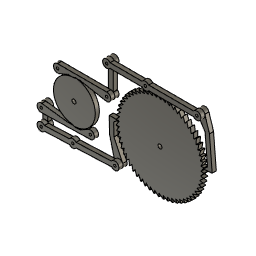
cam_driven_ratchet (Autodesk Fusion 360 design; units mm, degrees)
Autodesk Fusion 360 part; units mm, degrees
note: some values were not read from the file. Set by a fixed rule: which sketch regions a step uses.
sketch "dimensions" plane through (0, 0, 0) normal (0, 1, 0) x (1, 0, 0)
  circle A0 centre (0, 0) radius 25 construction
  line L0 (0, -25) -> (-20, -25) construction
  line L1 (0, -25) -> (40, -25) construction
  line L2 (40, -25) -> (40, -60) construction
  line L3 (40, -60) -> (87.1429, -60) construction
  line L4 (0, 25) -> (20, 25) construction
  line L5 (0, 25) -> (-40, 25) construction
  line L6 (-40, 25) -> (-40, 45) construction
  line L7 (-40, 45) -> (-1.4286, 45) construction
  line L8 (-1.4286, 45) -> (50, 45) construction
  line L9 (87.1429, -60) -> (150, -60) construction
  line L10 (50, 45) -> (50, 0) construction
  line L11 (150, -60) -> (150, 0) construction
  line L12 (150, 0) -> (50, 0) construction
  circle A1 centre (100, 0) radius 50 construction
  arc A2 (150, 0) -> (149.7261, 5.2264) centre (100, 0) ccw construction
  line L13 (100, 0) -> (150, 0) construction
  line L14 (100, 0) -> (149.7261, 5.2264) construction
  line L15 (0, 0) -> (300, 0) construction
  line L16 (0, -25) -> (0, -26) construction
  line L17 (-20, -25) -> (0, -26) construction
  line L18 (0, -26) -> (44.9579, -28.2479) construction
  line L19 (40, -25) -> (40, -28) construction
  arc A3 (39.9251, -27.9963) -> (40, -25) centre (-20, -25) ccw construction
  line L20 (-20, -25) -> (39.9251, -27.9963) construction
  line L21 (-20, -25) -> (40, -25) construction
  line L22 (40, -60) -> (40, -63) construction
  line L23 (150, -60) -> (150, -56) construction
  line L24 (40, -63) -> (150, -56) construction
  line L25 (0, 25) -> (0, 26) construction
  dimension "d4" = 20
  dimension "d5" = 40
  dimension "d6" = 35
  dimension "d7" = 47.1429
  dimension "d8" = 62.8571
  dimension "d9" = 20
  dimension "d10" = 40
  dimension "d11" = 20
  dimension "d12" = 38.5714
  dimension "d13" = 51.4286
  dimension "d14" = 50
  dimension "d25" = 100
  dimension "d173" = 6
  dimension "d185" = 1
  dimension "d190" = 3
  dimension "d191" = 2.862
  dimension "d192" = 3
  dimension "d193" = 4
  dimension "d195" = 1
  constraint coincident A0.centre L15.start
  constraint coincident A0 L0.start
  constraint horizontal L0
  constraint perpendicular L2 L3
  constraint coincident A0 L4.start
  constraint horizontal L4
  constraint perpendicular L5 L6
  constraint perpendicular L6 L7
  constraint parallel L7 L8
  constraint coincident L3.end L9.start
  constraint horizontal L3
  constraint horizontal L1
  constraint horizontal L5
  constraint tangent A0 L5
  constraint tangent A0 L1
  constraint perpendicular L9 L11
  constraint perpendicular L10 L12
  constraint midpoint L12 A1.centre
  constraint coincident L10.end A1
  constraint coincident A1.centre A2.centre
  constraint parallel L4 L15
  constraint collinear L12 L15
  constraint horizontal L9
  constraint parallel L17 L18
  constraint coincident L2 L19.end
  constraint coincident L18 L19.end
  constraint vertical L16
  constraint coincident L0.end L17.start
  constraint collinear L18 L20
  constraint perpendicular L3 L22
  constraint perpendicular L9 L23
  constraint perpendicular L4 L25
  measures "d4" distance of L0.start L0.end
  measures "d5" distance of L0.start L1.end
  measures "d6" distance of L1.end L2.end
  measures "d7" distance of L2.end L3.end
  measures "d8" distance of L3.end L9.end
  measures "d9" distance of L4.start L4.end
  measures "d10" distance of L4.start L5.end
  measures "d11" distance of L5.end L6.end
  measures "d12" distance of L6.end L7.end
  measures "d13" distance of L7.end L8.end
  measures "d14" diameter of A0
  measures "d25" diameter of A1
  measures "d173" angle of L13 L14
  measures "d185" distance of L0.start L16.end
  measures "d190" distance of L1.end L19.end
  measures "d191" angle of L20 L21
  measures "d192" distance of L2.end L22.end
  measures "d193" distance of L9.end L23.end
  measures "d195" distance of L4.start L25.end
sketch "cam" plane through (0, 0, 0) normal (0, 1, 0) x (1, 0, 0)
  circle A0 centre (0, 0) radius 2.5
  circle A1 centre (0, 0) radius 25 construction
  arc A2 (-1.3084, -24.9657) -> (0, -25) centre (0, 0) ccw construction
  line L0 (0, 0) -> (-1.3084, -24.9657) construction
  line L1 (0, 0) -> (0, -25) construction
  arc A3 (0, -26) -> (1.3607, -25.9644) centre (0, 0) ccw construction
  line L2 (0, 0) -> (0, -26) construction
  line L3 (0, 0) -> (1.3607, -25.9644) construction
  arc A4 (0, 25) -> (-1.3084, 24.9657) centre (0, 0) ccw construction
  line L4 (0, 0) -> (0, 25) construction
  line L5 (0, 0) -> (-1.3084, 24.9657) construction
  arc A5 (1.3607, 25.9644) -> (0, 26) centre (0, 0) ccw construction
  line L6 (0, 0) -> (1.3607, 25.9644) construction
  line L7 (0, 0) -> (0, 26) construction
  line L8 (-1.3084, 24.9657) -> (1.3607, 25.9644)
  line L9 (-1.3084, -24.9657) -> (1.3607, -25.9644)
  arc A6 (1.3607, -25.9644) -> (1.3607, 25.9644) centre (0, 0) ccw
  arc A7 (-1.3084, 24.9657) -> (-1.3084, -24.9657) centre (0, 0) ccw
  point P0 (0, -26)
  point P1 (0, -25)
  point P2 (0, 25)
  point P3 (0, 26)
  dimension "d194" = 5
  dimension "d196" = 3
  dimension "d197" = 3
  dimension "d198" = 3
  dimension "d199" = 3
  constraint coincident A0.centre A1.centre
  constraint coincident P1 A2.end
  constraint coincident P0 A3.start
  constraint coincident P2 A4.start
  constraint coincident P3 A5.end
  measures "d194" diameter of A0
  measures "d196" angle of L0 L1
  measures "d197" angle of L2 L3
  measures "d198" angle of L4 L5
  measures "d199" angle of L6 L7
sketch "arms" plane through (0, 0, 0) normal (0, 1, 0) x (1, 0, 0)
  circle A0 centre (20, 25) radius 1.5
  circle A1 centre (20, 25) radius 5
  circle A2 centre (-20, -25) radius 1.5
  circle A3 centre (-20, -25) radius 5
  circle A4 centre (-40, 25) radius 1.5
  circle A5 centre (-40, 45) radius 1.5
  circle A6 centre (-1.4286, 45) radius 1.5
  circle A7 centre (50, 45) radius 1.5
  circle A8 centre (40, -25) radius 1.5
  circle A9 centre (40, -60) radius 1.5
  circle A10 centre (87.1429, -60) radius 1.5
  circle A11 centre (150, -60) radius 1.5
  circle A12 centre (-40, 25) radius 5
  circle A13 centre (-40, 45) radius 5
  circle A14 centre (-1.4286, 45) radius 5
  circle A15 centre (50, 45) radius 5
  circle A16 centre (40, -25) radius 5
  circle A17 centre (40, -60) radius 5
  circle A18 centre (87.1429, -60) radius 5
  circle A19 centre (150, -60) radius 5
  line L0 (-1.3084, -24.9657) -> (-7.3084, -24.9657)
  line L1 (-7.3084, -24.9657) -> (-18.0426, -20.3991)
  line L2 (-20, -30) -> (40, -30)
  line L3 (20, 30) -> (-40, 30)
  line L4 (7.3607, -25.9644) -> (39.0888, -20.0837)
  line L5 (37, -60) -> (37, -25)
  line L6 (43, -60) -> (43, -25)
  line L7 (40, -63) -> (150, -63)
  line L8 (-1.3084, 24.9657) -> (-7.3084, 24.9657)
  line L9 (7.3607, 25.9644) -> (17.6839, 20.5688)
  line L10 (-7.3084, 24.9657) -> (-39.2405, 20.058)
  line L11 (1.3607, -25.9644) -> (7.3607, -25.9644)
  line L12 (1.3607, 25.9644) -> (7.3607, 25.9644)
  line L13 (-1.3084, -24.9657) -> (1.3607, -25.9644)
  line L14 (-1.3084, 24.9657) -> (1.3607, 25.9644)
  line L15 (-40, 25) -> (-43, 25) construction
  line L16 (-40, 25) -> (-37, 25) construction
  line L17 (-40, 45) -> (-43, 45) construction
  line L18 (-40, 45) -> (-37, 45) construction
  line L19 (-40, 45) -> (-40, 42) construction
  line L20 (-40, 45) -> (-40, 48) construction
  line L21 (50, 45) -> (50, 42) construction
  line L22 (50, 45) -> (50, 48) construction
  line L23 (40, -25) -> (43, -25) construction
  line L24 (40, -25) -> (37, -25) construction
  line L25 (40, -60) -> (37, -60) construction
  line L26 (40, -60) -> (43, -60) construction
  line L27 (40, -60) -> (40, -57) construction
  line L28 (40, -60) -> (40, -63) construction
  line L29 (150, -60) -> (150, -63) construction
  line L30 (150, -60) -> (150, -57) construction
  line L31 (150, -57) -> (40, -57)
  line L32 (-37, 25) -> (-37, 45)
  line L33 (-43, 25) -> (-43, 45)
  line L34 (-40, 42) -> (50, 42)
  line L35 (-40, 48) -> (50, 48)
  point P0 (40, -25)
  point P1 (-40, 25)
  point P2 (-40, 45)
  point P3 (40, -60)
  point P4 (150, -60)
  point P5 (50, 45)
  point P6 (-20, -25)
  point P7 (20, 25)
  point P8 (87.1429, -60)
  point P9 (-1.4286, 45)
  point P10 (-1.3084, 24.9657)
  point P11 (-1.3084, -24.9657)
  dimension "d37" = 3
  dimension "d38" = 10
  dimension "d39" = 3
  dimension "d40" = 10
  dimension "d41" = 3
  dimension "d42" = 3
  dimension "d43" = 3
  dimension "d44" = 3
  dimension "d45" = 3
  dimension "d46" = 3
  dimension "d47" = 3
  dimension "d48" = 3
  dimension "d49" = 10
  dimension "d50" = 10
  dimension "d51" = 10
  dimension "d52" = 10
  dimension "d53" = 10
  dimension "d54" = 10
  dimension "d55" = 10
  dimension "d56" = 10
  dimension "d57" = 6
  dimension "d149" = 6
  dimension "d170" = 6
  dimension "d171" = 6
  dimension "d200" = 3
  dimension "d201" = 3
  dimension "d203" = 3
  dimension "d204" = 3
  dimension "d205" = 3
  dimension "d206" = 3
  dimension "d207" = 3
  dimension "d208" = 3
  dimension "d209" = 3
  dimension "d210" = 3
  dimension "d211" = 3
  dimension "d212" = 3
  dimension "d213" = 3
  dimension "d214" = 3
  dimension "d215" = 3
  dimension "d216" = 3
  constraint coincident P7 A0.centre
  constraint concentric A0 A1
  constraint coincident P6 A2.centre
  constraint concentric A2 A3
  constraint coincident P1 A4.centre
  constraint coincident P2 A5.centre
  constraint coincident P9 A6.centre
  constraint coincident P5 A7.centre
  constraint coincident P0 A8.centre
  constraint coincident P3 A9.centre
  constraint coincident P8 A10.centre
  constraint coincident P4 A11.centre
  constraint concentric A4 A12
  constraint concentric A5 A13
  constraint concentric A8 A16
  constraint concentric A9 A17
  constraint concentric A11 A19
  constraint coincident A3 L1.end
  constraint tangent A3 L1
  constraint coincident A3 L2.start
  constraint coincident A16 L2.end
  constraint tangent A16 L2
  constraint horizontal L2
  constraint coincident A1 L3.start
  constraint coincident A12 L3.end
  constraint tangent A12 L3
  constraint parallel L2 L3
  constraint coincident A16 L4.end
  constraint tangent A16 L4
  constraint perpendicular L2 L5
  constraint perpendicular L2 L6
  constraint horizontal L7
  constraint horizontal L8
  constraint coincident A1 L9.end
  constraint tangent A1 L9
  constraint coincident A12 L10.end
  constraint tangent A12 L10
  constraint coincident L11.start L13.end
  constraint horizontal L11
  constraint coincident L4.start L11.end
  constraint coincident L12.start L14.end
  constraint horizontal L12
  constraint coincident L9.start L12.end
  constraint coincident P10 L8.start
  constraint coincident P11 L0.start
  constraint horizontal L0
  constraint parallel L3 L15
  constraint parallel L15 L16
  constraint horizontal L18
  constraint perpendicular L18 L19
  constraint perpendicular L18 L20
  constraint vertical L21
  constraint parallel L21 L22
  constraint perpendicular L6 L23
  constraint parallel L23 L24
  constraint perpendicular L5 L25
  constraint parallel L25 L26
  constraint perpendicular L26 L27
  constraint perpendicular L26 L28
  constraint coincident L5.start L25.end
  constraint coincident L5.end L24.end
  constraint coincident L6.end L23.end
  constraint coincident L6.start L26.end
  constraint coincident L7.start L28.end
  constraint vertical L29
  constraint parallel L29 L30
  constraint coincident L7.end L29.end
  constraint perpendicular L17 L33
  measures "d37" diameter of A0
  measures "d38" diameter of A1
  measures "d39" diameter of A2
  measures "d40" diameter of A3
  measures "d41" diameter of A4
  measures "d42" diameter of A5
  measures "d43" diameter of A6
  measures "d44" diameter of A7
  measures "d45" diameter of A8
  measures "d46" diameter of A9
  measures "d47" diameter of A10
  measures "d48" diameter of A11
  measures "d49" diameter of A12
  measures "d50" diameter of A13
  measures "d51" diameter of A14
  measures "d52" diameter of A15
  measures "d53" diameter of A16
  measures "d54" diameter of A17
  measures "d55" diameter of A18
  measures "d56" diameter of A19
  measures "d57" distance of P11 L0.end
  measures "d149" distance of P10 L8.end
  measures "d170" distance of L11.start L4.start
  measures "d171" distance of L12.start L9.start
  measures "d200" distance of P1 L15.end
  measures "d201" distance of P1 L16.end
  measures "d203" distance of P2 L17.end
  measures "d204" distance of P2 L18.end
  measures "d205" distance of P2 L19.end
  measures "d206" distance of P2 L20.end
  measures "d207" distance of P5 L21.end
  measures "d208" distance of P5 L22.end
  measures "d209" distance of P0 L6.end
  measures "d210" distance of P0 L5.end
  measures "d211" distance of P3 L5.start
  measures "d212" distance of P3 L6.start
  measures "d213" distance of P3 L27.end
  measures "d214" distance of P3 L7.start
  measures "d215" distance of P4 L7.end
  measures "d216" distance of P4 L30.end
sketch "pawls" plane through (0, 0, 0) normal (0, 1, 0) x (1, 0, 0)
  circle A0 centre (150, -60) radius 5
  circle A1 centre (150, -60) radius 1.5
  circle A2 centre (50, 45) radius 5
  circle A3 centre (50, 45) radius 1.5
  circle A4 centre (100, 0) radius 50 construction
  arc A5 (149.9315, -2.6168) -> (150, 0) centre (100, 0) ccw construction
  line L0 (100, 0) -> (149.9315, -2.6168) construction
  line L1 (100, 0) -> (150, 0) construction
  line L2 (149.9315, -2.6168) -> (153.9292, -2.7526)
  line L3 (153.9292, -2.7526) -> (160.9251, -2.9902)
  line L4 (153.9292, -2.7526) -> (153.8273, -5.7508) construction
  line L5 (149.9315, -2.6168) -> (153.8273, -5.7508)
  line L6 (153.8273, -5.7508) -> (155.3857, -7.0045)
  line L7 (160.9251, -2.9902) -> (159.5675, -42.9671)
  line L8 (159.5675, -42.9671) -> (154.8409, -61.2514)
  line L9 (159.5675, -42.9671) -> (148.1015, -42.5777) construction
  line L10 (155.3857, -7.0045) -> (154.1706, -42.7838)
  line L11 (154.1706, -42.7838) -> (145.6704, -57.499)
  line L12 (100, 0) -> (50, 0) construction
  line L13 (50, 0) -> (46, 0)
  line L14 (46, 0) -> (39, 0)
  line L15 (39, 0) -> (39, 20)
  line L16 (46, 0) -> (46, 3) construction
  line L17 (39, 20) -> (66.1936, 20) construction
  line L18 (50, 0) -> (46, 3)
  line L19 (44.4, 20) -> (54.572, 42.9759)
  line L20 (39, 20) -> (45.1321, 46.1419)
  line L21 (46, 3) -> (44.4, 4.2)
  line L22 (44.4, 4.2) -> (44.4, 20)
  dimension "d156" = 3
  dimension "d157" = 4
  dimension "d158" = 7
  dimension "d159" = 3
  dimension "d160" = 2
  dimension "d161" = 40
  dimension "d164" = 7
  dimension "d165" = 20
  dimension "d166" = 3
  dimension "d172" = 2
  dimension "d217" = 4
  constraint coincident A4 A5.end
  constraint coincident A4.centre A5.centre
  constraint parallel L2 L3
  constraint perpendicular L3 L4
  constraint parallel L5 L6
  constraint perpendicular L3 L7
  constraint coincident A0 L8.end
  constraint tangent A0 L8
  constraint perpendicular L7 L9
  constraint coincident L9 L10.end
  constraint perpendicular L9 L10
  constraint coincident A0 L11.end
  constraint tangent A0 L11
  constraint perpendicular L14 L15
  constraint perpendicular L14 L16
  constraint perpendicular L15 L17
  constraint coincident L17 L19.start
  constraint coincident A2 L19.end
  constraint tangent A2 L19
  constraint coincident A2 L20.end
  constraint tangent A2 L20
  constraint perpendicular L17 L22
  constraint coincident L19.start L22.end
  constraint horizontal L12
  constraint collinear L12 L13
  constraint coincident A4 L12.end
  constraint collinear L18 L21
  constraint horizontal L14
  constraint horizontal L1
  measures "d156" angle of L0 L1
  measures "d157" distance of A5.start L2.end
  measures "d158" distance of L2.end L3.end
  measures "d159" distance of L2.end L4.end
  measures "d160" distance of L4.end L6.end
  measures "d161" distance of L3.end L7.end
  measures "d164" distance of L13.end L14.end
  measures "d165" distance of L14.end L15.end
  measures "d166" distance of L13.end L16.end
  measures "d172" distance of L16.end L21.end
  measures "d217" distance of L12.end L13.end
sketch "wheel" plane through (0, 0, 0) normal (0, 1, 0) x (1, 0, 0)
  circle A0 centre (100, 0) radius 50 construction
  arc A1 (100, -50) -> (105.2264, -49.7261) centre (100, 0) ccw construction
  line L0 (100, 0) -> (100, -50) construction
  line L1 (100, 0) -> (105.2264, -49.7261) construction
  line L2 (100, -50) -> (100, -54)
  line L3 (100, -54) -> (105.2264, -49.7261)
  line L4 (105.6445, -53.7042) -> (110.3956, -48.9074)
  line L5 (105.2264, -49.7261) -> (105.6445, -53.7042)
  line L6 (111.2272, -52.82) -> (115.4508, -47.5528)
  line L7 (110.3956, -48.9074) -> (111.2272, -52.82)
  line L8 (116.6869, -51.3571) -> (120.3368, -45.6773)
  line L9 (115.4508, -47.5528) -> (116.6869, -51.3571)
  line L10 (121.9638, -49.3315) -> (125, -43.3013)
  line L11 (120.3368, -45.6773) -> (121.9638, -49.3315)
  line L12 (127, -46.7654) -> (129.3893, -40.4508)
  line L13 (125, -43.3013) -> (127, -46.7654)
  line L14 (131.7404, -43.6869) -> (133.4565, -37.1572)
  line L15 (129.3893, -40.4508) -> (131.7404, -43.6869)
  line L16 (136.1331, -40.1298) -> (137.1572, -33.4565)
  line L17 (133.4565, -37.1572) -> (136.1331, -40.1298)
  line L18 (140.1298, -36.1331) -> (140.4508, -29.3893)
  line L19 (137.1572, -33.4565) -> (140.1298, -36.1331)
  line L20 (143.6869, -31.7404) -> (143.3013, -25)
  line L21 (140.4508, -29.3893) -> (143.6869, -31.7404)
  line L22 (146.7654, -27) -> (145.6773, -20.3368)
  line L23 (143.3013, -25) -> (146.7654, -27)
  line L24 (149.3315, -21.9638) -> (147.5528, -15.4508)
  line L25 (145.6773, -20.3368) -> (149.3315, -21.9638)
  line L26 (151.3571, -16.6869) -> (148.9074, -10.3956)
  line L27 (147.5528, -15.4508) -> (151.3571, -16.6869)
  line L28 (152.82, -11.2272) -> (149.7261, -5.2264)
  line L29 (148.9074, -10.3956) -> (152.82, -11.2272)
  line L30 (153.7042, -5.6445) -> (150, 0)
  line L31 (149.7261, -5.2264) -> (153.7042, -5.6445)
  line L32 (154, 0) -> (149.7261, 5.2264)
  line L33 (150, 0) -> (154, 0)
  line L34 (153.7042, 5.6445) -> (148.9074, 10.3956)
  line L35 (149.7261, 5.2264) -> (153.7042, 5.6445)
  line L36 (152.82, 11.2272) -> (147.5528, 15.4508)
  line L37 (148.9074, 10.3956) -> (152.82, 11.2272)
  line L38 (151.3571, 16.6869) -> (145.6773, 20.3368)
  line L39 (147.5528, 15.4508) -> (151.3571, 16.6869)
  line L40 (149.3315, 21.9638) -> (143.3013, 25)
  line L41 (145.6773, 20.3368) -> (149.3315, 21.9638)
  line L42 (146.7654, 27) -> (140.4508, 29.3893)
  line L43 (143.3013, 25) -> (146.7654, 27)
  line L44 (143.6869, 31.7404) -> (137.1572, 33.4565)
  line L45 (140.4508, 29.3893) -> (143.6869, 31.7404)
  line L46 (140.1298, 36.1331) -> (133.4565, 37.1572)
  line L47 (137.1572, 33.4565) -> (140.1298, 36.1331)
  line L48 (136.1331, 40.1298) -> (129.3893, 40.4508)
  line L49 (133.4565, 37.1572) -> (136.1331, 40.1298)
  line L50 (131.7404, 43.6869) -> (125, 43.3013)
  line L51 (129.3893, 40.4508) -> (131.7404, 43.6869)
  line L52 (127, 46.7654) -> (120.3368, 45.6773)
  line L53 (125, 43.3013) -> (127, 46.7654)
  line L54 (121.9638, 49.3315) -> (115.4508, 47.5528)
  line L55 (120.3368, 45.6773) -> (121.9638, 49.3315)
  line L56 (116.6869, 51.3571) -> (110.3956, 48.9074)
  line L57 (115.4508, 47.5528) -> (116.6869, 51.3571)
  line L58 (111.2272, 52.82) -> (105.2264, 49.7261)
  line L59 (110.3956, 48.9074) -> (111.2272, 52.82)
  line L60 (105.6445, 53.7042) -> (100, 50)
  line L61 (105.2264, 49.7261) -> (105.6445, 53.7042)
  line L62 (100, 54) -> (94.7736, 49.7261)
  line L63 (100, 50) -> (100, 54)
  line L64 (94.3555, 53.7042) -> (89.6044, 48.9074)
  line L65 (94.7736, 49.7261) -> (94.3555, 53.7042)
  line L66 (88.7728, 52.82) -> (84.5492, 47.5528)
  line L67 (89.6044, 48.9074) -> (88.7728, 52.82)
  line L68 (83.3131, 51.3571) -> (79.6632, 45.6773)
  line L69 (84.5492, 47.5528) -> (83.3131, 51.3571)
  line L70 (78.0362, 49.3315) -> (75, 43.3013)
  line L71 (79.6632, 45.6773) -> (78.0362, 49.3315)
  line L72 (73, 46.7654) -> (70.6107, 40.4508)
  line L73 (75, 43.3013) -> (73, 46.7654)
  line L74 (68.2596, 43.6869) -> (66.5435, 37.1572)
  line L75 (70.6107, 40.4508) -> (68.2596, 43.6869)
  line L76 (63.8669, 40.1298) -> (62.8428, 33.4565)
  line L77 (66.5435, 37.1572) -> (63.8669, 40.1298)
  line L78 (59.8702, 36.1331) -> (59.5492, 29.3893)
  line L79 (62.8428, 33.4565) -> (59.8702, 36.1331)
  line L80 (56.3131, 31.7404) -> (56.6987, 25)
  line L81 (59.5492, 29.3893) -> (56.3131, 31.7404)
  line L82 (53.2346, 27) -> (54.3227, 20.3368)
  line L83 (56.6987, 25) -> (53.2346, 27)
  line L84 (50.6685, 21.9638) -> (52.4472, 15.4508)
  line L85 (54.3227, 20.3368) -> (50.6685, 21.9638)
  line L86 (48.6429, 16.6869) -> (51.0926, 10.3956)
  line L87 (52.4472, 15.4508) -> (48.6429, 16.6869)
  line L88 (47.18, 11.2272) -> (50.2739, 5.2264)
  line L89 (51.0926, 10.3956) -> (47.18, 11.2272)
  line L90 (46.2958, 5.6445) -> (50, 0)
  line L91 (50.2739, 5.2264) -> (46.2958, 5.6445)
  line L92 (46, 0) -> (50.2739, -5.2264)
  line L93 (50, 0) -> (46, 0)
  line L94 (46.2958, -5.6445) -> (51.0926, -10.3956)
  line L95 (50.2739, -5.2264) -> (46.2958, -5.6445)
  line L96 (47.18, -11.2272) -> (52.4472, -15.4508)
  line L97 (51.0926, -10.3956) -> (47.18, -11.2272)
  line L98 (48.6429, -16.6869) -> (54.3227, -20.3368)
  line L99 (52.4472, -15.4508) -> (48.6429, -16.6869)
  line L100 (50.6685, -21.9638) -> (56.6987, -25)
  line L101 (54.3227, -20.3368) -> (50.6685, -21.9638)
  line L102 (53.2346, -27) -> (59.5492, -29.3893)
  line L103 (56.6987, -25) -> (53.2346, -27)
  line L104 (56.3131, -31.7404) -> (62.8428, -33.4565)
  line L105 (59.5492, -29.3893) -> (56.3131, -31.7404)
  line L106 (59.8702, -36.1331) -> (66.5435, -37.1572)
  line L107 (62.8428, -33.4565) -> (59.8702, -36.1331)
  line L108 (63.8669, -40.1298) -> (70.6107, -40.4508)
  line L109 (66.5435, -37.1572) -> (63.8669, -40.1298)
  line L110 (68.2596, -43.6869) -> (75, -43.3013)
  line L111 (70.6107, -40.4508) -> (68.2596, -43.6869)
  line L112 (73, -46.7654) -> (79.6632, -45.6773)
  line L113 (75, -43.3013) -> (73, -46.7654)
  line L114 (78.0362, -49.3315) -> (84.5492, -47.5528)
  line L115 (79.6632, -45.6773) -> (78.0362, -49.3315)
  line L116 (83.3131, -51.3571) -> (89.6044, -48.9074)
  line L117 (84.5492, -47.5528) -> (83.3131, -51.3571)
  line L118 (88.7728, -52.82) -> (94.7736, -49.7261)
  line L119 (89.6044, -48.9074) -> (88.7728, -52.82)
  line L120 (94.3555, -53.7042) -> (100, -50)
  line L121 (94.7736, -49.7261) -> (94.3555, -53.7042)
  circle A2 centre (100, 0) radius 2.5
  line L122 (100, 0) -> (100, -50) construction
  point P0 (100, 0)
  dimension "d71" = 6
  dimension "d72" = 4
  dimension "d74" = 360
  dimension "d75" = 5
  constraint coincident A0 A1.start
  constraint coincident P0 A0.centre
  constraint parallel L0 L2
  constraint concentric A0 A2
  constraint vertical L122
  measures "d71" angle of L0 L1
  measures "d72" distance of A1.start L2.end
  measures "d75" diameter of A2
extrude "Extrude1" add sketch "cam" against normal blind 5 makes body 1 in component "cam"
extrude "Extrude1'" add sketch "arms" against normal blind 5 separate body contours A3 | A3 A16 L0 L1 L2 L4 L5 L11 L13 | A16 L2 L5 | A16 makes body 2 in component "push1"
extrude "Extrude1''" add sketch "arms" against normal blind 5 separate body contours A1 | A1 A12 L3 L8 L9 L10 L12 L14 L32 | A12 L3 L32 | A12 makes body 3 in component "push2"
extrude "Extrude1'''" add sketch "arms" along normal blind 5 separate body contours A16 L2 L5 | A16 A17 L2 L5 L6 | A16 | A17 L6 L31 | A17 L6 L31 makes body 4 in component "tie1"
extrude "Extrude1''''" add sketch "arms" along normal blind 5 separate body contours A12 L3 L32 | A12 A13 L3 L32 L33 | A12 | A13 L32 L34 | A13 L32 L34 makes body 5 in component "tie2"
extrude "Extrude1'''''" add sketch "arms" against normal blind 5 separate body contours A17 L6 L31 | A17 L6 L31 | A17 A18 L7 L31 | A18 L7 | A18 L7 L31 | A18 L31 | A18 A19 L7 L31 | A19 makes body 6 in component "arm1"
extrude "Extrude1''''''" add sketch "arms" against normal blind 5 separate body contours A13 L32 L34 | A13 L32 L34 | A13 A14 L34 L35 | A14 L34 | A14 L34 L35 | A14 L35 | A14 A15 L34 L35 | A15 makes body 7 in component "arm2"
extrude "Extrude1'''''''" add sketch "pawls" along normal blind 5 separate body contours A0 | A0 L2 L3 L5 L6 L7 L8 L10 L11 makes body 8 in component "pawl1"
extrude "Extrude1''''''''" add sketch "pawls" along normal blind 5 separate body contours A2 | A2 L13 L14 L15 L18 L19 L20 L21 L22 makes body 9 in component "pawl2"
extrude "Extrude1'''''''''" add sketch "wheel" along normal blind 5 separate body makes body 10 in component "wheel"
ref_plane "WorkPlane1" through (0, -10, 0) normal (0, 1, 0) x (0, 0, 1)
sketch "analysis" plane through (0, -10, 0) normal (0, 1, 0) x (1, 0, 0)
  circle A0 centre (100, 0) radius 50.9031 construction
  circle A1 centre (-1.4286, 45) radius 51.4286 construction
  line L0 (50, 45) -> (50, 0) construction
  line L1 (50, 45) -> (50, 41) construction
  line L2 (-1.4286, 45) -> (50, 41) construction
  line L3 (49.8451, 41.012) -> (49.253, -3.9841) construction
  line L4 (100, 0) -> (49.253, -3.9841)
  circle A2 centre (87.1429, -60) radius 62.8571 construction
  line L5 (150, -60) -> (150, -56) construction
  line L6 (87.1429, -60) -> (150, -56) construction
  line L7 (150, -60) -> (149.9315, -2.6168) construction
  line L8 (150.5543, -55.9647) -> (150.8834, 1.4173) construction
  line L9 (100, 0) -> (150.8834, 1.4173)
  line L10 (100, 0) -> (49.9811, -1.3932)
  arc A3 (150.7514, -3.9272) -> (150.8834, 1.4173) centre (100, 0) ccw construction
  line L11 (100, 0) -> (150.8834, 1.4173) construction
  line L12 (100, 0) -> (150.747, 3.9841) construction
  arc A4 (150.8854, -1.3423) -> (150.747, 3.9841) centre (100, 0) ccw construction
  line L13 (100, 0) -> (150.8854, -1.3423)
  line L14 (100, 0) -> (150.747, 3.9841) construction
  line L15 (50, 0) -> (150.9031, 0) construction
  line L16 (49.9811, -1.3932) -> (49.9811, 43.6068) construction
  arc A5 (49.9811, 43.6068) -> (50, 45) centre (-1.4286, 45) ccw construction
  line L17 (-1.4286, 45) -> (49.9811, 43.6068) construction
  line L18 (-1.4286, 45) -> (50, 45) construction
  arc A6 (49.8451, 41.012) -> (50, 45) centre (-1.4286, 45) ccw
  line L19 (-1.4286, 45) -> (49.8451, 41.012) construction
  line L20 (-1.4286, 45) -> (50, 45) construction
  line L21 (150.8854, -1.3423) -> (149.9869, -58.7182) construction
  arc A7 (150, -60) -> (149.9869, -58.7182) centre (87.1429, -60) ccw construction
  line L22 (87.1429, -60) -> (150, -60) construction
  line L23 (87.1429, -60) -> (149.9869, -58.7182) construction
  arc A8 (150, -60) -> (149.8704, -55.9656) centre (87.1429, -60) ccw construction
  line L24 (87.1429, -60) -> (150, -60) construction
  line L25 (87.1429, -60) -> (149.8704, -55.9656) construction
  point P0 (-1.4286, 45)
  point P1 (49.0969, 0.0091)
  point P2 (50, 45)
  point P3 (100, 0)
  point P4 (87.1429, -60)
  point P5 (150, -60)
  point P6 (100, 0)
  point P7 (149.9315, -2.6168)
  point P8 (150.5543, -55.9647)
  dimension "d220" = 45
  dimension "d221" = 4
  dimension "d222" = 45
  dimension "d224" = 4
  dimension "d225" = 57.3832
  dimension "d226" = 57.383
  dimension "d228" = 6
  dimension "d231" = 45
  dimension "d232" = 1.552
  dimension "d233" = 4.447
  dimension "d234" = 57.383
  dimension "d235" = 1.168
  dimension "d236" = 3.68
  constraint coincident P6 P3
  constraint coincident P1 A0
  constraint coincident P0 A1.centre
  constraint coincident P2 A1
  constraint coincident P2 L0.start
  constraint vertical L0
  constraint parallel L0 L1
  constraint coincident A1 L3.start
  constraint coincident L2 L3.start
  constraint coincident A0 L3.end
  constraint coincident P4 A2.centre
  constraint coincident P5 A2
  constraint coincident P5 L5.start
  constraint vertical L5
  constraint coincident P7 L7.end
  constraint coincident L6 P8
  constraint coincident P8 L8.start
  constraint coincident A0 L8.end
  constraint collinear L9 L10
  constraint coincident A0 L12.end
  constraint collinear L4 L12
  constraint coincident A3 L15.end
  constraint parallel L1 L16
  constraint coincident L3.start A6.start
  constraint coincident A2 L21.end
  constraint coincident L21.end A7.end
  measures "d220" distance of P2 L0.end
  measures "d221" distance of P2 L1.end
  measures "d222" distance of L3.start L3.end
  measures "d224" distance of P5 L5.end
  measures "d225" vertical distance of P5 P7
  measures "d226" distance of P8 L8.end
  measures "d228" angle of L13 L14
  measures "d231" distance of L10.end L16.end
  measures "d232" angle of L17 L18
  measures "d233" angle of L19 L20
  measures "d234" distance of A4.start L21.end
  measures "d235" angle of L22 L23
  measures "d236" angle of L24 L25
component "cam" placed x (1, 0, 0) y (0, 1, 0) z (0, 0, 1) at (0, 0, 0)
component "push1" placed x (1, 0, 0) y (0, 1, 0) z (0, 0, 1) at (0, 0, 0)
component "push2" placed x (1, 0, 0) y (0, 1, 0) z (0, 0, 1) at (0, 0, 0)
component "tie1" placed x (1, 0, 0) y (0, 1, 0) z (0, 0, 1) at (0, 0, 0)
component "tie2" placed x (1, 0, 0) y (0, 1, 0) z (0, 0, 1) at (0, 0, 0)
component "arm1" placed x (1, 0, 0) y (0, 1, 0) z (0, 0, 1) at (0, 0, 0)
component "arm2" placed x (1, 0, 0) y (0, 1, 0) z (0, 0, 1) at (0, 0, 0)
component "pawl1" placed x (0.998789, 0, 0.049198) y (0, 1, 0) z (-0.049198, 0, 0.998789) at (3.1336, 0, -7.3071)
component "pawl2" placed x (0.999799, 0, 0.02007) y (0, 1, 0) z (-0.02007, 0, 0.999799) at (-0.8931, 0, -1.0126)
component "wheel" placed x (0.999657, 0, 0.026177) y (0, 1, 0) z (-0.026177, 0, 0.999657) at (0.0343, 0, -2.6177)
component "ground" placed x (1, 0, 0) y (0, 1, 0) z (0, 0, 1) at (0, 0, 0)
equation "d7 = ( 3 * 110 / 7 ) * 1 mm"
equation "d8 = ( 4 * 110 / 7 ) * 1 mm"
equation "d12 = ( 3 * 90 / 7 ) * 1 mm"
equation "d13 = ( 4 * 90 / 7 ) * 1 mm"
